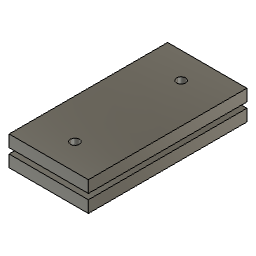
floorcowl_flat v7 (Autodesk Fusion 360 design; units mm, degrees)
Autodesk Fusion 360 part; units mm, degrees
sketch "Sketch1" plane through (0, 0, 0) normal (0, 1, 0) x (1, 0, 0)
  line L0 (0, 0) -> (25.4, 0)
  line L1 (25.4, 0) -> (25.4, -3.81)
  line L2 (25.4, -3.81) -> (0, -3.81)
  line L3 (0, -3.81) -> (0, 0)
  line L4 (0, -3.81) -> (25.4, -3.81) construction
  line L5 (25.4, -3.81) -> (25.4, -5.5626) construction
  line L6 (25.4, -5.5626) -> (0, -5.5626) construction
  line L7 (0, -5.5626) -> (0, -3.81) construction
  line L8 (25.4, -5.5626) -> (0, -5.5626)
  line L9 (0, -5.5626) -> (0, -9.3726)
  line L10 (0, -9.3726) -> (25.4, -9.3726)
  line L11 (25.4, -9.3726) -> (25.4, -5.5626)
  dimension "d1" = 25.4
  dimension "d2" = 3.81
  dimension "d3" = 25.4
  dimension "d4" = 1.7526
  dimension "d5" = 3.81
  constraint horizontal L0
  constraint vertical L1
  constraint horizontal L2
  constraint vertical L3
  constraint coincident L0.start L3.end
  constraint horizontal L4
  constraint vertical L5
  constraint horizontal L6
  constraint vertical L7
  constraint perpendicular L8 L9
  constraint parallel L8 L10
  constraint parallel L9 L11
  measures "d1" distance of L0.start L0.end
  measures "d2" distance of L0.start L2.end
  measures "d3" distance of L2.end L1.end
  measures "d4" distance of L2.end L6.end
  measures "d5" distance of L5.end L10.end
extrude "Extrude1" add sketch "Sketch1" along normal blind 50.8 makes body 1 at (8.4667, 33.8667, 9.3726) makes body 2 at (16.9333, 33.8667, 3.81)
sketch "Sketch2" plane through (0, 0, 9.3726) normal (0, 0, 1) x (-1, 0, 0)
  line L0 (0, 0) -> (-25.4, 0)
  line L1 (-25.4, 0) -> (-25.4, -50.8)
  line L2 (-25.4, -50.8) -> (0, -50.8)
  line L3 (0, -50.8) -> (0, 0)
  line L4 (-25.4, -50.8) -> (0, -50.8) construction
  line L5 (0, -50.8) -> (0, 0) construction
  line L6 (0, 0) -> (-25.4, 0) construction
  line L7 (-25.4, 0) -> (-25.4, -50.8) construction
  line L8 (-12.7, -50.8) -> (-12.7, 0)
  point P0 (-12.7, -25.4)
  point P1 (-12.7, -42.418)
  point P2 (-12.7, -8.382)
  dimension "d13" = 8.382
  dimension "d14" = 8.382
  constraint horizontal L4
  constraint vertical L5
  constraint horizontal L6
  constraint vertical L7
  constraint coincident L0.start L3.end
  constraint coincident L1.end L2.start
  constraint midpoint L2 L8.start
  constraint midpoint L0 L8.end
  constraint midpoint L8 P0
  constraint coincident L8 P1
  constraint coincident L8 P2
  measures "d13" distance of L4 P1
  measures "d14" distance of L8.end P2
hole "Hole1" at (12.7, 42.418, 9.3726) at (12.7, 8.382, 9.3726) direction (0, 0, -1) diameter 2.8702 depth 10.16 tip angle 180 bodies 1 2
